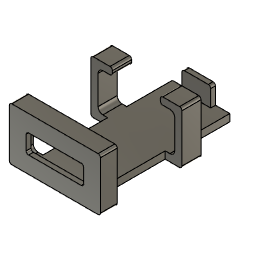
Collin_Battery_Holder_Square v2 v2 (Autodesk Fusion 360 design; units mm, degrees)
Autodesk Fusion 360 part; units mm, degrees
note: some values were not read from the file. Chosen so that the rebuilt part matches the saved one: which face or edge a step refers to.
sketch "Sketch1" plane through (0, 0, 0) normal (0, 1, 0) x (1, 0, 0)
  line L0 (0, 0) -> (38, 0)
  line L1 (38, 0) -> (38, -22)
  line L2 (38, -22) -> (0, -22)
  line L3 (0, -22) -> (0, 0)
  line L4 (3, -3) -> (35, -3)
  line L5 (35, -3) -> (35, -19)
  line L6 (35, -19) -> (3, -19)
  line L7 (3, -19) -> (3, -3)
  line L8 (7, -3) -> (31, -3)
  line L9 (31, -3) -> (31, 0)
  line L10 (31, 0) -> (7, 0)
  line L11 (7, 0) -> (7, -3)
  line L12 (9, -22) -> (29, -22)
  line L13 (29, -22) -> (29, -19)
  line L14 (29, -19) -> (9, -19)
  line L15 (9, -19) -> (9, -22)
  circle A0 centre (19, -25.5) radius 3.05
  circle A1 centre (19, -25.5) radius 5
  line L16 (0, -11) -> (38, -11)
  circle A2 centre (19, 3.5) radius 3.05
  circle A3 centre (19, 3.5) radius 5
  line L17 (7, -15) -> (31, -15)
  line L18 (31, -15) -> (31, -7)
  line L19 (31, -7) -> (7, -7)
  line L20 (7, -7) -> (7, -15)
  dimension "d1" = 38
  dimension "d2" = 22
  dimension "d4" = 32
  dimension "d5" = 16
  dimension "d6" = 3
  dimension "d7" = 3
  dimension "d8" = 24
  dimension "d9" = 7
  dimension "d16" = 9
  dimension "d17" = 9
  dimension "d26" = 6.1
  dimension "d27" = 19
  dimension "d28" = 3.5
  dimension "d29" = 10
  dimension "d37" = 4
  dimension "d38" = 4
  dimension "d39" = 4
  dimension "d40" = 4
  constraint horizontal L0
  constraint vertical L1
  constraint horizontal L2
  constraint vertical L3
  constraint coincident L0.start L3.end
  constraint horizontal L4
  constraint vertical L5
  constraint horizontal L6
  constraint vertical L7
  constraint horizontal L8
  constraint vertical L9
  constraint horizontal L10
  constraint vertical L11
  constraint coincident L4 L8.start
  constraint collinear L0 L10
  constraint horizontal L12
  constraint vertical L13
  constraint horizontal L14
  constraint vertical L15
  constraint coincident L6 L13.end
  constraint coincident L2 L12.start
  constraint concentric A0 A1
  constraint midpoint L3 L16.start
  constraint midpoint L1 L16.end
  constraint symmetric A0 L16 A2
  constraint symmetric A1 L16 A3
  constraint horizontal L17
  constraint vertical L18
  constraint horizontal L19
  constraint vertical L20
  measures "d1" distance of L0.start L0.end
  measures "d2" distance of L0.end L1.end
  measures "d4" distance of L5 L7
  measures "d5" distance of L4 L6
  measures "d6" distance of L0 L4
  measures "d7" distance of L3 L7
  measures "d8" distance of L9 L11
  measures "d9" distance of L3 L11
  measures "d16" distance of L3 L15
  measures "d17" distance of L1 L13
  measures "d26" diameter of A0
  measures "d27" distance of L1 A0.centre
  measures "d28" distance of L2 A0.centre
  measures "d29" diameter of A1
  measures "d37" distance of L6 L17
  measures "d38" distance of L5 L18
  measures "d39" distance of L4 L19
  measures "d40" distance of L7 L20
extrude "Extrude1" add sketch "Sketch1" along normal blind 3 contours L0 L3 L4 L7 L11 L16 | L0 L4 L8 L9 L10 L11 A3 | L2 L3 L6 L7 L15 L16 | L0 L10 A3 | L4 L5 L7 L8 L16 L18 L19 L20 | L5 L6 L7 L14 L16 L17 L18 L20 | L0 L1 L4 L5 L9 L16 | L2 L6 L12 L13 L14 L15 A1 | L16 L18 L19 L20 | L16 L17 L18 L20 | L2 L12 A1 | L1 L2 L5 L6 L13 L16 picked at (17.9903, -0.1594) picked at (19.3587, -21.5391)
extrude "Extrude2" add sketch "Sketch1" along normal blind 63 contours L0 L4 L8 L9 L10 L11 A3 | L0 L10 A3 picked at (17.9903, -0.1594)
extrude "Extrude3" add sketch "Sketch1" along normal blind 8 contours L0 L3 L4 L7 L11 L16 | L2 L3 L6 L7 L15 L16 | L0 L1 L4 L5 L9 L16 | L2 L6 L12 L13 L14 L15 A1 | L2 L12 A1 | L1 L2 L5 L6 L13 L16 picked at (19.3587, -21.5391)
extrude "Extrude4" add sketch "Sketch1" along normal blind 8 from surface at 35 contours L0 L3 L4 L7 L11 L16 | L2 L3 L6 L7 L15 L16 | L0 L1 L4 L5 L9 L16 | L1 L2 L5 L6 L13 L16
sketch "Sketch2" plane through (0, 0, 3) normal (0, 0, 1) x (-1, 0, 0)
  line L0 (-3, -3) -> (-35, -3)
  line L1 (-35, -3) -> (-35, -8)
  line L2 (-35, -8) -> (-31, -8)
  line L3 (-31, -8) -> (-31, -35)
  line L4 (-31, -35) -> (-35, -35)
  line L5 (-35, -35) -> (-35, -43)
  line L6 (-35, -43) -> (-31, -43)
  line L7 (-31, -43) -> (-31, -63)
  line L8 (-31, -63) -> (-7, -63)
  line L9 (-7, -63) -> (-7, -43)
  line L10 (-7, -43) -> (-3, -43)
  line L11 (-3, -43) -> (-3, -35)
  line L12 (-3, -35) -> (-7, -35)
  line L13 (-7, -35) -> (-7, -8)
  line L14 (-7, -8) -> (-3, -8)
  line L15 (-3, -8) -> (-3, -3)
  line L16 (-13, -63) -> (-25, -63)
  line L17 (-25, -63) -> (-25, -60)
  line L18 (-25, -60) -> (-13, -60)
  line L19 (-13, -60) -> (-13, -63)
  dimension "d21" = 3
  dimension "d22" = 6
  dimension "d23" = 6
  constraint horizontal L16
  constraint vertical L17
  constraint horizontal L18
  constraint vertical L19
  constraint coincident L8 L16.start
  measures "d21" distance of L16.end L17.end
  measures "d22" distance of L7 L17
  measures "d23" distance of L9 L19
extrude "Extrude5" add sketch "Sketch2" along normal blind 8 contours L8 L16 L17 L18 L19
extrude "Extrude6" [suppressed]
fillet "Fillet1" radius 1 14 edges at (38, 4, 22) (0, 4, 22) (38, 39, 22) (0, 39, 22) (38, 4, 0) (0, 4, 0) (13, 61.5, 11) (25, 61.5, 11) (0, 39, 0) (38, 39, 0) (29, 39, 22) (29, 39, 19) (9, 39, 19) (9, 39, 22) 1 faces at (13.6667, 3, 8.3333)
fillet "Fillet2" radius 2 12 edges at (3, 39, 19) (35, 39, 19) (3, 39, 3) (35, 39, 3) (34.7071, 3.2929, 3.2929) (35, 6, 3) (3.2929, 3.2929, 3.2929) (3, 6, 3) (3.2929, 3.2929, 18.7071) (3, 6, 19) (34.7071, 3.2929, 18.7071) (35, 6, 19)
extrude "Extrude7" cut sketch "Sketch1" along normal blind 3 contours L16 L18 L19 L20 | L16 L17 L18 L20
fillet "Fillet3" radius 1 4 edges at (31, 1.5, 15) (31, 1.5, 7) (7, 1.5, 7) (7, 1.5, 15)
extrude "Extrude8" cut 1 faces at (15.3333, 0, 2.3333) along direction (0, 1, 0) blind 1
extrude "Extrude9" cut 1 faces at (17.3333, 63, 5.6667) along direction (0, -1, 0) blind 1
ref_plane "WorkPlane2" through (19, 31.5, 11) normal (0, -1, 0) x (-1, 0, 0)
sketch "Sketch4" plane through (19, 31.5, 11) normal (0, -1, 0) x (1, 0, 0)
  arc A0 (2.4575, -15.7207) -> (-2.4575, -15.7207) centre (0, -14) ccw
  line L0 (-12, -11) -> (12, -11)
  line L1 (0, -14) -> (0, -11)
  line L2 (0, -14) -> (-2.4575, -15.7207) construction
  line L3 (0, -14) -> (-3, -14) construction
  arc A1 (-2.4575, -19.1622) -> (-2.4575, -15.7207) centre (-4.9149, -17.4415) ccw
  arc A2 (2.4575, -15.7207) -> (2.4575, -19.1622) centre (4.9149, -17.4415) ccw
  dimension "d56" = 35
  dimension "d57" = 3
  dimension "d58" = 3
  dimension "d59" = 3
  constraint coincident A0.centre L1.start
  constraint midpoint L0 L1.end
  constraint vertical L1
  constraint coincident A0 L3.end
  constraint perpendicular L1 L3
  constraint symmetric A0.start A0.end L1
  constraint vertical A0.end A1.start
  constraint tangent A0 A1
  constraint symmetric A0.end L1 A0.start
  constraint symmetric L1 A1.start A2.end
  constraint symmetric L1 A1 A2
  measures "d56" angle of L2 L3
  measures "d57" radius of A1
  measures "d58" radius of A0
  measures "d59" distance of A0.centre L1.end
extrude "Extrude11" add sketch "Sketch4" along normal mid plane 24 thin wall 1 on the left open curves A1 A0 A2
fillet "Fillet4" radius 0.5 2 edges at (21.4575, 31.5, -8.1622) (22.2766, 31.5, -7.5886)
fillet "Fillet4" radius 0.5 2 edges at (15.7234, 31.5, -7.5886) (16.5425, 31.5, -8.1622)
fillet "Fillet5" radius 0.8 2 edges at (16.3542, 31.5, 0) (21.6458, 31.5, 0)
equation "d1 = 30 mm + 6 mm + 2 mm"
equation "d2 = 14 mm + 6 mm + 2 mm"
equation "d9 = ( ( 38 - 24 ) / 2 ) * 1 mm"
equation "d12 = 3 mm + 55 mm + 3 mm + 2 mm"
equation "d14 = 3 mm + 5 mm"
equation "d27 = 7 mm + ( 24 / 2 ) * 1 mm"
equation "d57 = d58"
